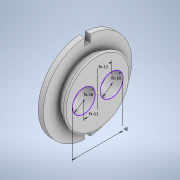
# Autodesk Inventor part: SpacerCorrect
Saved by Autodesk Inventor 2021.2 (Build 252289000, 289)
## iProperties
Created: 2023-01-30
Part Number: SpacerCorrect
Material: Типовые
Document SubType Name: Modeling
Designer: Andrei
Density: 1 g/cm^3
Appearance: По умолчанию
Author: Andrei
Autodesk Inventor part; units mm, degrees
ref_plane "YZ Plane" through (0, 0, 0) normal (1, 0, 0) x (0, 1, 0)
ref_plane "XZ Plane" through (0, 0, 0) normal (0, 1, 0) x (-1, 0, 0)
ref_plane "XY Plane" through (0, 0, 0) normal (0, 0, 1) x (1, 0, 0)
sketch "Эскиз1" plane through (0, 0, 0) normal (0, 0, 1) x (1, 0, 0)
  line L0 (0, 0) -> (4, 0)
  line L1 (4, 0) -> (4, -35)
  line L2 (4, -35) -> (0, -35)
  line L3 (0, -35) -> (0, 0)
  line L4 (4, 0) -> (12, 0)
  line L5 (12, 0) -> (12, -24.8868)
  line L6 (12, -26.6188) -> (4, -26.6188)
  line L7 (4, -26.6188) -> (4, 0)
  line L8 (4, 0) -> (4, -22)
  line L9 (4, -22) -> (10.5, -25.7528)
  arc A0 (10.5, -25.7528) -> (12, -24.8868) centre (11, -24.8868) ccw
  dimension "d0" = 4
  dimension "d1" = 35
  dimension "d2" = 8
  dimension "d4" = 22
  dimension "d36" = 60
  dimension "d37" = 1
  constraints: 20 end point, 4 parallel, 3 point on line, 2 horizontal, 2 perpendicular, 2 point on circle, 2 tangent, 1 centre point
  measures "d0" distance of L1.end L2.end
  measures "d1" distance of L0.end L1.end
  measures "d2" distance of L6.start L6.end
  measures "d4" distance of L0.end L8.end
  measures "d36" angle of L9 L1
  measures "d37" radius of A0
revolve "Вращение1" add sketch "Эскиз1" angle 360 about axis through (0, 0, 0) along (1, 0, 0)
mirror "Зеркальное отражение1" [suppressed]
sketch "Эскиз2" plane through (12, 0, 0) normal (1, 0, 0) x (0, 0, -1)
  circle A0 centre (11, 0) radius 9
  circle A1 centre (-11, 0) radius 9
  point P0 (0, 0)
  dimension "d6" = 18
  dimension "d7" = 18
  dimension "d8" = 11
  dimension "d9" = 11
  dimension "d10" = 40
  constraints: 2 centre point
  measures "d6" diameter of A0
  measures "d7" diameter of A1
  measures "d8" distance of A0.centre point (0, 0)
  measures "d9" distance of A1.centre point (0, 0)
hole "Отверстие1" at (12, 0, 11) direction (-1, 0, 0) diameter 18 end through all
hole "Отверстие2" at (12, 0, -11) direction (-1, 0, 0) diameter 18 end through all
sketch "Эскиз3" plane through (4, 0, 0) normal (1, 0, 0) x (0, 0, -1)
  line L0 (-2.25, 35) -> (2.25, 35)
  line L1 (2.25, 35) -> (2.25, 29.3705)
  line L2 (2.25, 29.3705) -> (-2.25, 29.3705)
  line L3 (-2.25, 29.3705) -> (-2.25, 35)
  circle A0 centre (0, 0) radius 35 projected
  line L4 (0, 35) -> (0, 30.5)
  line L5 (0, -35) -> (0, -30.5)
  line L6 (-2.25, -30.5) -> (2.25, -30.5)
  line L7 (2.25, -30.5) -> (2.25, -35)
  line L8 (2.25, -35) -> (-2.25, -35)
  line L9 (-2.25, -35) -> (-2.25, -30.5)
  point P0 (0, 0)
  dimension "d25" = 4.5
  dimension "d26" = 4.5
  dimension "d27" = 2.25
  dimension "d28" = 0
  dimension "d29" = 4.5
  dimension "d30" = 4.5
  dimension "d31" = 4.5
  dimension "d32" = 2.25
  dimension "d33" = 0
  constraints: 20 end point, 4 parallel, 2 horizontal, 2 perpendicular, 2 point on circle, 2 vertical
  measures "d25" distance of L1.end L2.end
  measures "d26" distance of L4.start L4.end
  measures "d27" distance between parallel lines of L4 L3
  measures "d28" distance from line of L4.start L0
  measures "d29" distance of L5.start L5.end
  measures "d30" distance of L6.end L7.end
  measures "d31" distance of L6.start L6.end
  measures "d32" distance between parallel lines of L5 L9
  measures "d33" distance from line of L5.end L6
extrude "Выдавливание1" cut sketch "Эскиз3" against normal blind 4 contours L0 A0 L3 | L0 L1 A0 | A0 L1 L2 L3 | L9 L6 L5 A0 | A0 L8 L9 | L5 L6 L7 A0 | A0 L7 L8
equation "\"d0\" = 0.5 * hFlange"
equation "\"d1\" = 0.5 * dOuter"
equation "\"d2\" = hMount"
equation "\"d4\" = 0.5 * dMinimal"
equation "\"d36\" = angleMount"
equation "\"d6\" = dHoles"
equation "\"d7\" = dHoles"
equation "\"d8\" = r2holes"
equation "\"d9\" = r2holes"
equation "\"d11\" = dHoles"
equation "\"d18\" = dHoles"
equation "\"d25\" = wSlot"
equation "\"d26\" = hSlot"
equation "\"d27\" = 0.5 * wSlot"
equation "\"d29\" = hSlot"
equation "\"d30\" = hSlot"
equation "\"d31\" = wSlot"
equation "\"d32\" = 0.5 * wSlot"
equation "\"hFlange\" = 8"
equation "\"dMinimal\" = 44"
equation "\"angleMount\" = 60deg"
equation "\"dHoles\" = 18"
equation "\"r2holes\" = 11"
equation "\"hMount\" = 8"
equation "\"wSlot\" = 4.5"
equation "\"hSlot\" = 4.5"
equation "\"dOuter\" = 70"
